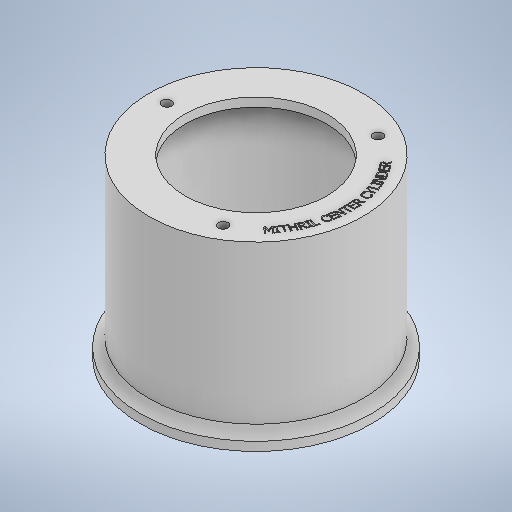
# Autodesk Inventor part: Mithril Center Cylinder
Saved by Autodesk Inventor 2026.2 (Build 302298000, 298)
## iProperties
Created: 2026-03-06
Part Number: Mithril Center Cylinder
Material: Generic
Document SubType Name: Modeling
Designer: mumin
Density: 1 g/cm^3
Appearance: Default
Author: mumin
Autodesk Inventor part; units mm, degrees
note: some values were not read from the file. Chosen so that the rebuilt part matches the saved one: direction of "Hole1".
ref_plane "YZ Plane" through (0, 0, 0) normal (1, 0, 0) x (0, 1, 0)
ref_plane "XZ Plane" through (0, 0, 0) normal (0, 1, 0) x (-1, 0, 0)
ref_plane "XY Plane" through (0, 0, 0) normal (0, 0, 1) x (1, 0, 0)
sketch "Sketch1" plane through (0, 0, 0) normal (1, 0, 0) x (0, 1, 0)
  line L0 (0, 0) -> (100, 0)
  line L1 (100, -40.5) -> (95, -40.5)
  line L2 (95, -40.5) -> (95, -56)
  line L3 (95, -56) -> (0, -56)
  line L4 (0, -56) -> (0, -66)
  line L5 (0, -66) -> (5, -66)
  line L6 (5, -66) -> (5, -61)
  line L7 (5, -61) -> (100, -61)
  line L8 (100, -61) -> (100, -40.5)
  line L9 (5, -66) -> (9.9531, -61)
  point P0 (97.5, -40.5)
  dimension "d0" = 100
  dimension "d1" = 81
  dimension "d2" = 122
  dimension "d3" = 100
  dimension "d4" = 5
  dimension "d5" = 5
  dimension "d6" = 5
  dimension "d7" = 10
  constraints: 20 end point, 7 perpendicular, 2 horizontal, 2 point on line, 1 midpoint
  measures "d0" distance of L0.start L0.end
  measures "d1" diameter of point (97.5, -40.5) L0
  measures "d2" diameter of L7 L0
  measures "d3" distance between parallel lines of L4 L8
  measures "d4" distance between parallel lines of L2 L8
  measures "d5" distance between parallel lines of L4 L6
  measures "d6" distance between parallel lines of L7 L3
  measures "d7" distance between parallel lines of L5 L3
revolve "Revolution1" add sketch "Sketch1" angle 360 about axis through (0, 0, 0) along (0, 1, 0)
sketch "Sketch2" plane through (0, 100, 0) normal (0, 1, 0) x (1, 0, 0)
  circle A0 centre (0, 0) radius 51
  point P0 (-51, 0)
  point P1 (25.5, -44.1673)
  point P2 (25.5, 44.1673)
  dimension "d9" = 102
  dimension "d12" = 360
  constraints: 1 coincident, 1 horizontal alignment, 6 other
hole "Hole1" at (-51, 100, 0) at (25.5, 100, 44.1673) at (25.5, 100, -44.1673) direction (0, -1, 0) diameter 5.5 end up to surface
sketch "Sketch3" plane through (0, 100, 0) normal (0, 1, 0) x (1, 0, 0)
  circle A0 centre (25.5, 44.1673) radius 2.75 projected
  circle A1 centre (25.5, -44.1673) radius 2.75 projected
  circle A2 centre (-51, 0) radius 2.75 projected
  circle A3 centre (0, 0) radius 40.5 projected
  circle A4 centre (0, 0) radius 61 projected
  line L0 (43.7454, -33.3925) -> (43.3661, -33.8549)
  line L1 (43.3661, -33.8549) -> (40.3691, -31.3962)
  line L2 (40.3691, -31.3962) -> (41.6628, -33.9763)
  line L3 (41.6628, -33.9763) -> (41.4315, -34.2582)
  line L4 (41.4315, -34.2582) -> (38.6553, -33.4854)
  line L5 (38.6553, -33.4854) -> (41.6522, -35.944)
  line L6 (41.6522, -35.944) -> (41.2984, -36.3754)
  line L7 (41.2984, -36.3754) -> (37.8193, -33.5212)
  line L8 (37.8193, -33.5212) -> (38.3374, -32.8897)
  line L9 (38.3374, -32.8897) -> (40.9866, -33.6103)
  line L10 (40.9866, -33.6103) -> (39.739, -31.1812)
  line L11 (39.739, -31.1812) -> (40.2664, -30.5384)
  line L12 (40.2664, -30.5384) -> (43.7454, -33.3925)
  line L13 (45.1833, -31.3723) -> (44.1667, -32.7883)
  line L14 (44.1667, -32.7883) -> (43.7934, -32.5203)
  line L15 (43.7934, -32.5203) -> (44.1273, -32.0552)
  line L16 (44.1273, -32.0552) -> (41.2185, -29.9666)
  line L17 (41.2185, -29.9666) -> (40.8846, -30.4316)
  line L18 (40.8846, -30.4316) -> (40.5113, -30.1636)
  line L19 (40.5113, -30.1636) -> (41.528, -28.7477)
  line L20 (41.528, -28.7477) -> (41.9012, -29.0157)
  line L21 (41.9012, -29.0157) -> (41.5673, -29.4808)
  line L22 (41.5673, -29.4808) -> (44.4762, -31.5694)
  line L23 (44.4762, -31.5694) -> (44.8101, -31.1043)
  line L24 (44.8101, -31.1043) -> (45.1833, -31.3723)
  line L25 (46.175, -29.8824) -> (42.8323, -27.7451)
  line L26 (42.8323, -27.7451) -> (42.0191, -29.0171)
  line L27 (42.0191, -29.0171) -> (41.5705, -28.7303)
  line L28 (41.5705, -28.7303) -> (43.5192, -25.6825)
  line L29 (43.5192, -25.6825) -> (43.9677, -25.9693)
  line L30 (43.9677, -25.9693) -> (43.1545, -27.2413)
  line L31 (43.1545, -27.2413) -> (46.4972, -29.3785)
  line L32 (46.4972, -29.3785) -> (46.175, -29.8824)
  line L33 (49.0995, -24.8376) -> (48.8139, -25.363)
  line L34 (48.8139, -25.363) -> (46.8788, -24.3108)
  line L35 (46.8788, -24.3108) -> (45.8894, -26.1305)
  line L36 (45.8894, -26.1305) -> (47.8244, -27.1827)
  line L37 (47.8244, -27.1827) -> (47.5387, -27.7081)
  line L38 (47.5387, -27.7081) -> (43.5853, -25.5585)
  line L39 (43.5853, -25.5585) -> (43.871, -25.0331)
  line L40 (43.871, -25.0331) -> (45.4216, -25.8762)
  line L41 (45.4216, -25.8762) -> (46.4111, -24.0565)
  line L42 (46.4111, -24.0565) -> (44.8605, -23.2134)
  line L43 (44.8605, -23.2134) -> (45.1462, -22.688)
  line L44 (45.1462, -22.688) -> (49.0995, -24.8376)
  line L45 (50.9362, -20.8466) -> (50.6158, -21.5542)
  line L46 (50.6158, -21.5542) -> (48.3981, -22.1112)
  line L47 (48.3981, -22.1112) -> (48.1153, -22.7358)
  line L48 (48.1153, -22.7358) -> (49.7464, -23.4743)
  line L49 (49.7464, -23.4743) -> (49.4998, -24.0191)
  line L50 (49.4998, -24.0191) -> (45.4004, -22.163)
  line L51 (45.4004, -22.163) -> (45.8787, -21.1066)
  spline S0 degree 2 poles (45.8787, -21.1066) (46.0381, -20.7545) (46.3296, -20.314) (46.5669, -20.1613) knots 0 0 0 1 2 2 2
  spline S1 degree 2 poles (46.5669, -20.1613) (46.8042, -20.0085) (47.3522, -19.9564) (47.6744, -20.1023) knots 0 0 0 1 2 2 2
  spline S2 degree 2 poles (47.6744, -20.1023) (48.1229, -20.3054) (48.5233, -21.039) (48.4919, -21.4972) knots 0 0 0 1 2 2 2
  line L52 (48.4919, -21.4972) -> (50.9362, -20.8466)
  spline S3 degree 2 poles (47.4604, -20.6899) (47.281, -20.6087) (46.9481, -20.6101) (46.7983, -20.7024) knots 0 0 0 1 2 2 2
  spline S4 degree 2 poles (46.7983, -20.7024) (46.6692, -20.784) (46.4662, -21.0644) (46.3639, -21.2903) knots 0 0 0 1 2 2 2
  line L53 (46.3639, -21.2903) -> (46.1188, -21.8318)
  line L54 (46.1188, -21.8318) -> (47.6602, -22.5297)
  line L55 (47.6602, -22.5297) -> (47.8768, -22.0513)
  spline S5 degree 2 poles (47.8768, -22.0513) (47.9836, -21.8155) (48.0705, -21.4025) (47.9996, -21.2143) knots 0 0 0 1 2 2 2
  spline S6 degree 2 poles (47.9996, -21.2143) (47.9408, -21.0435) (47.673, -20.7862) (47.4604, -20.6899) knots 0 0 0 1 2 2 2
  line L56 (51.6063, -19.0406) -> (50.9771, -20.6663)
  line L57 (50.9771, -20.6663) -> (50.5486, -20.5004)
  line L58 (50.5486, -20.5004) -> (50.7553, -19.9665)
  line L59 (50.7553, -19.9665) -> (47.4156, -18.6739)
  line L60 (47.4156, -18.6739) -> (47.209, -19.2079)
  line L61 (47.209, -19.2079) -> (46.7805, -19.042)
  line L62 (46.7805, -19.042) -> (47.4097, -17.4164)
  line L63 (47.4097, -17.4164) -> (47.8382, -17.5823)
  line L64 (47.8382, -17.5823) -> (47.6315, -18.1162)
  line L65 (47.6315, -18.1162) -> (50.9711, -19.4087)
  line L66 (50.9711, -19.4087) -> (51.1778, -18.8748)
  line L67 (51.1778, -18.8748) -> (51.6063, -19.0406)
  line L68 (52.6823, -15.8712) -> (51.8613, -18.3459)
  line L69 (51.8613, -18.3459) -> (47.5902, -16.929)
  line L70 (47.5902, -16.929) -> (47.7786, -16.3614)
  line L71 (47.7786, -16.3614) -> (51.5443, -17.6107)
  line L72 (51.5443, -17.6107) -> (52.177, -15.7036)
  line L73 (52.177, -15.7036) -> (52.6823, -15.8712)
  spline S7 degree 2 poles (53.7897, -11.8585) (53.6928, -12.2852) (53.2407, -12.9416) (52.8929, -13.1393) knots 0 0 0 1 2 2 2
  spline S8 degree 2 poles (52.8929, -13.1393) (52.5486, -13.3378) (51.6297, -13.4319) (51.0749, -13.3058) knots 0 0 0 1 2 2 2
  spline S9 degree 2 poles (51.0749, -13.3058) (50.5238, -13.1806) (49.7697, -12.7138) (49.528, -12.3784) knots 0 0 0 1 2 2 2
  spline S10 degree 2 poles (49.528, -12.3784) (49.2927, -12.0482) (49.1465, -11.2596) (49.2476, -10.8151) knots 0 0 0 1 2 2 2
  spline S11 degree 2 poles (49.2476, -10.8151) (49.2977, -10.5946) (49.4497, -10.2216) (49.5367, -10.0693) knots 0 0 0 1 2 2 2
  spline S12 degree 2 poles (49.5367, -10.0693) (49.6152, -9.9376) (49.8139, -9.6723) (49.9253, -9.5443) knots 0 0 0 1 2 2 2
  line L74 (49.9253, -9.5443) -> (50.6293, -9.7043)
  line L75 (50.6293, -9.7043) -> (50.6188, -9.7505)
  spline S13 degree 2 poles (50.6188, -9.7505) (50.5299, -9.8126) (50.2759, -10.0091) (50.1403, -10.1616) knots 0 0 0 1 2 2 2
  spline S14 degree 2 poles (50.1403, -10.1616) (50.0098, -10.3077) (49.8028, -10.6757) (49.7446, -10.9318) knots 0 0 0 1 2 2 2
  spline S15 degree 2 poles (49.7446, -10.9318) (49.6808, -11.2127) (49.798, -11.7666) (49.9756, -12.0052) knots 0 0 0 1 2 2 2
  spline S16 degree 2 poles (49.9756, -12.0052) (50.1576, -12.241) (50.7899, -12.6016) (51.2131, -12.6978) knots 0 0 0 1 2 2 2
  spline S17 degree 2 poles (51.2131, -12.6978) (51.6647, -12.8004) (52.3648, -12.7313) (52.6316, -12.5938) knots 0 0 0 1 2 2 2
  spline S18 degree 2 poles (52.6316, -12.5938) (52.8906, -12.4582) (53.2234, -12.014) (53.2864, -11.7366) knots 0 0 0 1 2 2 2
  spline S19 degree 2 poles (53.2864, -11.7366) (53.3438, -11.4841) (53.3171, -11.0256) (53.2626, -10.8374) knots 0 0 0 1 2 2 2
  spline S20 degree 2 poles (53.2626, -10.8374) (53.2065, -10.6564) (53.0686, -10.3745) (53.0164, -10.2916) knots 0 0 0 1 2 2 2
  line L76 (53.0164, -10.2916) -> (53.0261, -10.2489)
  line L77 (53.0261, -10.2489) -> (53.7231, -10.4073)
  spline S21 degree 2 poles (53.7231, -10.4073) (53.7575, -10.5684) (53.8238, -10.8528) (53.8395, -11.047) knots 0 0 0 1 2 2 2
  spline S22 degree 2 poles (53.8395, -11.047) (53.8599, -11.2536) (53.8495, -11.5953) (53.7897, -11.8585) knots 0 0 0 1 2 2 2
  line L78 (54.1123, -9.9247) -> (49.6684, -9.2161)
  line L79 (49.6684, -9.2161) -> (50.1117, -6.436)
  line L80 (50.1117, -6.436) -> (50.6375, -6.5198)
  line L81 (50.6375, -6.5198) -> (50.2884, -8.7093)
  line L82 (50.2884, -8.7093) -> (51.5056, -8.9034)
  line L83 (51.5056, -8.9034) -> (51.8312, -6.8616)
  line L84 (51.8312, -6.8616) -> (52.3569, -6.9454)
  line L85 (52.3569, -6.9454) -> (52.0313, -8.9873)
  line L86 (52.0313, -8.9873) -> (53.6807, -9.2503)
  line L87 (53.6807, -9.2503) -> (54.0298, -7.0608)
  line L88 (54.0298, -7.0608) -> (54.5556, -7.1446)
  line L89 (54.5556, -7.1446) -> (54.1123, -9.9247)
  line L90 (54.9253, -3.2867) -> (54.8657, -3.955)
  line L91 (54.8657, -3.955) -> (50.8239, -5.5932)
  line L92 (50.8239, -5.5932) -> (54.6886, -5.9382)
  line L93 (54.6886, -5.9382) -> (54.639, -6.4939)
  line L94 (54.639, -6.4939) -> (50.1568, -6.0938)
  line L95 (50.1568, -6.0938) -> (50.2324, -5.2475)
  line L96 (50.2324, -5.2475) -> (53.9422, -3.7591)
  line L97 (53.9422, -3.7591) -> (50.3935, -3.4423)
  line L98 (50.3935, -3.4423) -> (50.4431, -2.8866)
  line L99 (50.4431, -2.8866) -> (54.9253, -3.2867)
  line L100 (54.9848, -1.3264) -> (51.0179, -1.2525)
  line L101 (51.0179, -1.2525) -> (50.9898, -2.762)
  line L102 (50.9898, -2.762) -> (50.4575, -2.7521)
  line L103 (50.4575, -2.7521) -> (50.5249, 0.8648)
  line L104 (50.5249, 0.8648) -> (51.0572, 0.8549)
  line L105 (51.0572, 0.8549) -> (51.0291, -0.6546)
  line L106 (51.0291, -0.6546) -> (54.996, -0.7284)
  line L107 (54.996, -0.7284) -> (54.9848, -1.3264)
  line L108 (55.0009, 1.24) -> (50.5056, 1.034)
  line L109 (50.5056, 1.034) -> (50.3767, 3.8462)
  line L110 (50.3767, 3.8462) -> (50.9086, 3.8706)
  line L111 (50.9086, 3.8706) -> (51.0101, 1.6558)
  line L112 (51.0101, 1.6558) -> (52.2414, 1.7122)
  line L113 (52.2414, 1.7122) -> (52.1467, 3.7777)
  line L114 (52.1467, 3.7777) -> (52.6786, 3.8021)
  line L115 (52.6786, 3.8021) -> (52.7732, 1.7366)
  line L116 (52.7732, 1.7366) -> (54.4417, 1.8131)
  line L117 (54.4417, 1.8131) -> (54.3401, 4.0279)
  line L118 (54.3401, 4.0279) -> (54.872, 4.0523)
  line L119 (54.872, 4.0523) -> (55.0009, 1.24)
  line L120 (54.4277, 8.1668) -> (54.5147, 7.3949)
  line L121 (54.5147, 7.3949) -> (52.8948, 5.7811)
  line L122 (52.8948, 5.7811) -> (52.9716, 5.0998)
  line L123 (52.9716, 5.0998) -> (54.7509, 5.3004)
  line L124 (54.7509, 5.3004) -> (54.8178, 4.7061)
  line L125 (54.8178, 4.7061) -> (50.3462, 4.202)
  line L126 (50.3462, 4.202) -> (50.2163, 5.3544)
  spline S23 degree 2 poles (50.2163, 5.3544) (50.173, 5.7385) (50.1979, 6.2661) (50.3235, 6.5188) knots 0 0 0 1 2 2 2
  spline S24 degree 2 poles (50.3235, 6.5188) (50.4492, 6.7715) (50.8933, 7.0968) (51.2448, 7.1364) knots 0 0 0 1 2 2 2
  spline S25 degree 2 poles (51.2448, 7.1364) (51.734, 7.1915) (52.4535, 6.7662) (52.6611, 6.3566) knots 0 0 0 1 2 2 2
  line L127 (52.6611, 6.3566) -> (54.4277, 8.1668)
  spline S26 degree 2 poles (51.3617, 6.522) (51.166, 6.5) (50.8808, 6.3284) (50.7993, 6.1724) knots 0 0 0 1 2 2 2
  spline S27 degree 2 poles (50.7993, 6.1724) (50.7302, 6.0362) (50.6994, 5.6914) (50.7272, 5.445) knots 0 0 0 1 2 2 2
  line L128 (50.7272, 5.445) -> (50.7937, 4.8543)
  line L129 (50.7937, 4.8543) -> (52.4752, 5.0439)
  line L130 (52.4752, 5.0439) -> (52.4163, 5.5657)
  spline S28 degree 2 poles (52.4163, 5.5657) (52.3873, 5.823) (52.2506, 6.2222) (52.0933, 6.3476) knots 0 0 0 1 2 2 2
  spline S29 degree 2 poles (52.0933, 6.3476) (51.9554, 6.4642) (51.5936, 6.5482) (51.3617, 6.522) knots 0 0 0 1 2 2 2
  spline S30 degree 2 poles (53.7234, 12.1552) (53.8172, 11.7278) (53.6874, 10.9414) (53.4568, 10.6145) knots 0 0 0 1 2 2 2
  spline S31 degree 2 poles (53.4568, 10.6145) (53.2297, 10.2884) (52.4381, 9.8123) (51.8825, 9.6903) knots 0 0 0 1 2 2 2
  spline S32 degree 2 poles (51.8825, 9.6903) (51.3304, 9.5691) (50.4494, 9.6707) (50.088, 9.8714) knots 0 0 0 1 2 2 2
  spline S33 degree 2 poles (50.088, 9.8714) (49.7345, 10.0701) (49.2667, 10.7216) (49.169, 11.1668) knots 0 0 0 1 2 2 2
  spline S34 degree 2 poles (49.169, 11.1668) (49.1205, 11.3877) (49.0994, 11.79) (49.1133, 11.9648) knots 0 0 0 1 2 2 2
  spline S35 degree 2 poles (49.1133, 11.9648) (49.1284, 12.1174) (49.1953, 12.442) (49.2416, 12.6052) knots 0 0 0 1 2 2 2
  line L131 (49.2416, 12.6052) -> (49.9468, 12.76)
  line L132 (49.9468, 12.76) -> (49.957, 12.7137)
  spline S36 degree 2 poles (49.957, 12.7137) (49.903, 12.6197) (49.7566, 12.3337) (49.6988, 12.1381) knots 0 0 0 1 2 2 2
  spline S37 degree 2 poles (49.6988, 12.1381) (49.6429, 11.9503) (49.6122, 11.5292) (49.6684, 11.2727) knots 0 0 0 1 2 2 2
  spline S38 degree 2 poles (49.6684, 11.2727) (49.7302, 10.9913) (50.0719, 10.5399) (50.3342, 10.3996) knots 0 0 0 1 2 2 2
  spline S39 degree 2 poles (50.3342, 10.3996) (50.5993, 10.2636) (51.3249, 10.2064) (51.7488, 10.2994) knots 0 0 0 1 2 2 2
  spline S40 degree 2 poles (51.7488, 10.2994) (52.2012, 10.3987) (52.8053, 10.759) (52.9883, 10.9971) knots 0 0 0 1 2 2 2
  spline S41 degree 2 poles (52.9883, 10.9971) (53.1649, 11.23) (53.2771, 11.7735) (53.2161, 12.0514) knots 0 0 0 1 2 2 2
  spline S42 degree 2 poles (53.2161, 12.0514) (53.1606, 12.3043) (52.9413, 12.7079) (52.812, 12.855) knots 0 0 0 1 2 2 2
  spline S43 degree 2 poles (52.812, 12.855) (52.6842, 12.9949) (52.4395, 13.1914) (52.3569, 13.2442) knots 0 0 0 1 2 2 2
  line L133 (52.3569, 13.2442) -> (52.3475, 13.2869)
  line L134 (52.3475, 13.2869) -> (53.0457, 13.4401)
  spline S44 degree 2 poles (53.0457, 13.4401) (53.1454, 13.309) (53.3264, 13.0799) (53.4232, 12.9107) knots 0 0 0 1 2 2 2
  spline S45 degree 2 poles (53.4232, 12.9107) (53.5296, 12.7325) (53.6656, 12.4188) (53.7234, 12.1552) knots 0 0 0 1 2 2 2
  line L135 (47.9939, 15.8123) -> (50.8276, 15.0524)
  line L136 (50.8276, 15.0524) -> (52.7395, 15.6082)
  line L137 (52.7395, 15.6082) -> (52.9064, 15.0339)
  line L138 (52.9064, 15.0339) -> (51.054, 14.4955)
  line L139 (51.054, 14.4955) -> (49.0098, 12.3176)
  line L140 (49.0098, 12.3176) -> (48.8245, 12.9549)
  line L141 (48.8245, 12.9549) -> (50.4012, 14.6247)
  line L142 (50.4012, 14.6247) -> (48.171, 15.203)
  line L143 (48.171, 15.203) -> (47.9939, 15.8123)
  line L144 (51.2648, 19.9811) -> (52.144, 17.5264)
  line L145 (52.144, 17.5264) -> (47.9076, 16.009)
  line L146 (47.9076, 16.009) -> (47.7059, 16.5721)
  line L147 (47.7059, 16.5721) -> (51.4411, 17.9099)
  line L148 (51.4411, 17.9099) -> (50.7636, 19.8016)
  line L149 (50.7636, 19.8016) -> (51.2648, 19.9811)
  line L150 (50.4762, 21.8611) -> (51.1436, 20.2508)
  line L151 (51.1436, 20.2508) -> (50.7191, 20.0749)
  line L152 (50.7191, 20.0749) -> (50.4999, 20.6038)
  line L153 (50.4999, 20.6038) -> (47.1917, 19.2327)
  line L154 (47.1917, 19.2327) -> (47.411, 18.7038)
  line L155 (47.411, 18.7038) -> (46.9865, 18.5279)
  line L156 (46.9865, 18.5279) -> (46.3191, 20.1382)
  line L157 (46.3191, 20.1382) -> (46.7436, 20.3141)
  line L158 (46.7436, 20.3141) -> (46.9628, 19.7852)
  line L159 (46.9628, 19.7852) -> (50.271, 21.1563)
  line L160 (50.271, 21.1563) -> (50.0517, 21.6852)
  line L161 (50.0517, 21.6852) -> (50.4762, 21.8611)
  line L162 (48.7882, 25.4422) -> (49.0809, 24.8385)
  line L163 (49.0809, 24.8385) -> (46.4581, 21.3542)
  line L164 (46.4581, 21.3542) -> (49.9495, 23.0468)
  line L165 (49.9495, 23.0468) -> (50.1929, 22.5448)
  line L166 (50.1929, 22.5448) -> (46.1437, 20.5817)
  line L167 (46.1437, 20.5817) -> (45.773, 21.3462)
  line L168 (45.773, 21.3462) -> (48.1883, 24.5313)
  line L169 (48.1883, 24.5313) -> (44.9823, 22.9771)
  line L170 (44.9823, 22.9771) -> (44.7389, 23.4791)
  line L171 (44.7389, 23.4791) -> (48.7882, 25.4422)
  spline S46 degree 2 poles (44.6348, 28.1836) (45.1674, 28.4936) (46.276, 28.5608) (46.7265, 28.3377) knots 0 0 0 1 2 2 2
  spline S47 degree 2 poles (46.7265, 28.3377) (47.0849, 28.1497) (47.565, 27.6148) (47.8401, 27.142) knots 0 0 0 1 2 2 2
  line L172 (47.8401, 27.142) -> (48.3611, 26.2469)
  line L173 (48.3611, 26.2469) -> (44.4719, 23.9833)
  line L174 (44.4719, 23.9833) -> (43.9564, 24.8689)
  spline S48 degree 2 poles (43.9564, 24.8689) (43.6373, 25.4173) (43.4379, 26.1368) (43.4545, 26.4418) knots 0 0 0 1 2 2 2
  spline S49 degree 2 poles (43.4545, 26.4418) (43.4852, 26.9617) (44.0675, 27.8534) (44.6348, 28.1836) knots 0 0 0 1 2 2 2
  spline S50 degree 2 poles (44.9422, 27.641) (44.4946, 27.3805) (44.0336, 26.7155) (44.0245, 26.3178) knots 0 0 0 1 2 2 2
  spline S51 degree 2 poles (44.0245, 26.3178) (44.0227, 26.0383) (44.1857, 25.5045) (44.3893, 25.1546) knots 0 0 0 1 2 2 2
  line L175 (44.3893, 25.1546) -> (44.6186, 24.7607)
  line L176 (44.6186, 24.7607) -> (47.6127, 26.5033)
  line L177 (47.6127, 26.5033) -> (47.3834, 26.8973)
  spline S52 degree 2 poles (47.3834, 26.8973) (47.1835, 27.2408) (46.7705, 27.6967) (46.4995, 27.8216) knots 0 0 0 1 2 2 2
  spline S53 degree 2 poles (46.4995, 27.8216) (46.1589, 27.9863) (45.396, 27.9051) (44.9422, 27.641) knots 0 0 0 1 2 2 2
  line L178 (46.2122, 29.8509) -> (42.49, 27.3219)
  line L179 (42.49, 27.3219) -> (40.9079, 29.6505)
  line L180 (40.9079, 29.6505) -> (41.3483, 29.9497)
  line L181 (41.3483, 29.9497) -> (42.5943, 28.1158)
  line L182 (42.5943, 28.1158) -> (43.6138, 28.8085)
  line L183 (43.6138, 28.8085) -> (42.4518, 30.5187)
  line L184 (42.4518, 30.5187) -> (42.8922, 30.818)
  line L185 (42.8922, 30.818) -> (44.0542, 29.1077)
  line L186 (44.0542, 29.1077) -> (45.4357, 30.0463)
  line L187 (45.4357, 30.0463) -> (44.1896, 31.8803)
  line L188 (44.1896, 31.8803) -> (44.63, 32.1795)
  line L189 (44.63, 32.1795) -> (46.2122, 29.8509)
  line L190 (42.0975, 35.4524) -> (42.5757, 34.8404)
  line L191 (42.5757, 34.8404) -> (42.0404, 32.6173)
  line L192 (42.0404, 32.6173) -> (42.4625, 32.0771)
  line L193 (42.4625, 32.0771) -> (43.8734, 33.1794)
  line L194 (43.8734, 33.1794) -> (44.2416, 32.7082)
  line L195 (44.2416, 32.7082) -> (40.6956, 29.9376)
  line L196 (40.6956, 29.9376) -> (39.9816, 30.8514)
  spline S54 degree 2 poles (39.9816, 30.8514) (39.7437, 31.156) (39.4887, 31.6186) (39.4634, 31.8997) knots 0 0 0 1 2 2 2
  spline S55 degree 2 poles (39.4634, 31.8997) (39.4382, 32.1808) (39.6463, 32.6904) (39.925, 32.9082) knots 0 0 0 1 2 2 2
  spline S56 degree 2 poles (39.925, 32.9082) (40.3129, 33.2113) (41.1486, 33.2256) (41.54, 32.9853) knots 0 0 0 1 2 2 2
  line L197 (41.54, 32.9853) -> (42.0975, 35.4524)
  spline S57 degree 2 poles (40.3463, 32.446) (40.1911, 32.3247) (40.0379, 32.0292) (40.0501, 31.8536) knots 0 0 0 1 2 2 2
  spline S58 degree 2 poles (40.0501, 31.8536) (40.0626, 31.7014) (40.2168, 31.3915) (40.3695, 31.1961) knots 0 0 0 1 2 2 2
  line L198 (40.3695, 31.1961) -> (40.7354, 30.7277)
  line L199 (40.7354, 30.7277) -> (42.0688, 31.7695)
  line L200 (42.0688, 31.7695) -> (41.7455, 32.1833)
  spline S59 degree 2 poles (41.7455, 32.1833) (41.5861, 32.3873) (41.2605, 32.6559) (41.0609, 32.6804) knots 0 0 0 1 2 2 2
  spline S60 degree 2 poles (41.0609, 32.6804) (40.8824, 32.7075) (40.5302, 32.5897) (40.3463, 32.446) knots 0 0 0 1 2 2 2
  constraints: 1 other
emboss "Emboss1" sketch "Sketch3" operation cut depth 1 direction (0, -1, 0) contours L0 L1 L2 L3 L4 L5 L6 L7 L8 L9 L10 L11 L12 | L13 L14 L15 L16 L17 L18 L19 L20 L21 L22 L23 L24 | L25 L26 L27 L28 L29 L30 L31 L32 | L33 L34 L35 L36 L37 L38 L39 L40 L41 L42 L43 L44 | L45 L46 L47 L48 L49 L50 L51 S0 S1 S2 L52 | L56 L57 L58 L59 L60 L61 L62 L63 L64 L65 L66 L67 | L68 L69 L70 L71 L72 L73 | S7 S8 S9 S10 S11 S12 L74 L75 S13 S14 S15 S16 S17 S18 S19 S20 L76 L77 S21 S22 | L78 L79 L80 L81 L82 L83 L84 L85 L86 L87 L88 L89 | L90 L91 L92 L93 L94 L95 L96 L97 L98 L99 | L100 L101 L102 L103 L104 L105 L106 L107 | L108 L109 L110 L111 L112 L113 L114 L115 L116 L117 L118 L119 | L120 L121 L122 L123 L124 L125 L126 S23 S24 S25 L127 | S30 S31 S32 S33 S34 S35 L139 L131 L132 S36 S37 S38 S39 S40 S41 S42 S43 L133 L134 S44 S45 | L139 L140 L141 L142 L143 L135 L136 L137 L138 L131 S35 | S35 L131 L139 | L144 L145 L146 L147 L148 L149 | L150 L151 L152 L153 L154 L155 L156 L157 L158 L159 L160 L161 | L162 L163 L164 L165 L166 L167 L168 L169 L170 L171 | S46 S47 L172 L173 L174 S48 S49 | L178 L179 L180 L181 L182 L183 L184 L185 L186 L187 L188 L189 | L190 L191 L192 L193 L194 L195 L196 S54 S55 S56 L197
body "Solid1"
